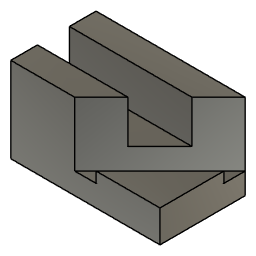
que5 v1 (Autodesk Fusion 360 design; units mm, degrees)
Autodesk Fusion 360 part; units mm, degrees
sketch "Sketch1" plane through (0, 0, 0) normal (0, 0, 1) x (1, 0, 0)
  line L0 (0, 0) -> (70, 0)
  line L1 (70, 0) -> (70, 40)
  line L2 (70, 40) -> (0, 40)
  line L3 (0, 40) -> (0, 0)
  dimension "d1" = 70
  dimension "d2" = 40
  constraint horizontal L0
  constraint vertical L1
  constraint horizontal L2
  constraint vertical L3
  constraint coincident L0.start L3.end
  measures "d1" distance of L0.start L0.end
  measures "d2" distance of L0.start L2.end
extrude "Extrude1" add sketch "Sketch1" along normal blind 15 makes body 1
sketch "Sketch2" plane through (0, 0, 15) normal (0, 0, 1) x (-1, 0, 0)
  line L0 (0, -40) -> (0, 0)
  line L1 (0, 0) -> (-70, 0)
  line L2 (-70, 0) -> (-70, -40)
  line L3 (-70, -40) -> (0, -40)
  line L4 (0, -27.5) -> (-70, -27.5)
  line L5 (0, -12.5) -> (-70, -12.5)
  dimension "d5" = 12.5
  dimension "d6" = 12.5
  constraint coincident L0 L4.start
  constraint coincident L2 L4.end
  constraint perpendicular L2 L4
  constraint coincident L0 L5.start
  constraint coincident L2 L5.end
  constraint perpendicular L2 L5
  measures "d5" distance of L3 L4
  measures "d6" distance of L1 L5
extrude "Extrude2" add sketch "Sketch2" along normal blind 25 contours L0 L2 L3 L4 bodies 1
extrude "Extrude3" add sketch "Sketch2" along normal blind 25 contours L0 L1 L2 L5 bodies 1
move_face "MoveFace1" by (0, 0, 5) 1 faces at (23.3333, 17.5, 15) on bodies 1
box "BoxPrimitive1" add length 40 width 40 height 40 placed x (0, 0, -1) y (0, 1, 0) z (1, 0, 0) at (0, -93.9243, 42.2229) separate body makes body 2
chamfer "Chamfer1" distance 40 distance2 40 1 edges at (0, -53.9243, 22.2229) measured on face at (0, -67.2577, 28.8896) on bodies 2
move_body "Move1" bodies 2 to x (1, 0, 0) y (0, 1, 0) z (0, 0, 1) at (30, 94, 0)
move_face "MoveFace2" by (0, 0, 10) 2 faces at (56.664, 13.4117, 42.2229) (56.664, 13.4117, 2.2229) on bodies 2
move_body "Move2" bodies 2 to x (1, 0, 0) y (0, 1, 0) z (0, 0, 1) at (0, 0, -12)
move_body "Move3" bodies 2 to x (1, 0, 0) y (0, 1, 0) z (0, 0, 1) at (0, -0.0757, -0.2229)
move_face "MoveFace3" by (0, 0, 10) 1 faces at (56.664, 13.336, 0) on bodies 2
combine "Combine1" operation cut target body 1 tool bodies 2
sketch "Sketch4" plane through (0, 0, 10) normal (0, 0, 1) x (-1, 0, 0)
  line L0 (-70, -40) -> (-30, 0)
  line L1 (-30, 0) -> (-70, 0)
  line L2 (-70, 0) -> (-70, -40)
  line L3 (-40, 0) -> (-70, -30)
  line L4 (0, -40) -> (0, -27.5)
  dimension "d33" = 30
  dimension "d34" = 30
  dimension "d35" = 70
  constraint coincident L1 L3.start
  measures "d33" distance of L1.end L3.end
  measures "d34" distance of L1.end L3.start
  measures "d35" distance of L3.end L4
extrude "Extrude4" add sketch "Sketch4" along normal blind 5 contours L1 L2 L3 bodies 1
